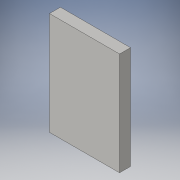
# Autodesk Inventor part: cwbreadboard
Saved by Autodesk Inventor 2016 (Build 200138000, 138)
## iProperties
Created: 2017-08-31
Part Number: cwbreadboard
Material: Generic
Document SubType Name: Modeling
Designer: student
Density: 1 g/cm^3
Appearance: Default
Author: student
Autodesk Inventor part; units mm, degrees
ref_plane "YZ Plane" through (0, 0, 0) normal (1, 0, 0) x (0, 1, 0)
ref_plane "XZ Plane" through (0, 0, 0) normal (0, 1, 0) x (-1, 0, 0)
ref_plane "XY Plane" through (0, 0, 0) normal (0, 0, 1) x (1, 0, 0)
sketch "Sketch1" plane through (0, 0, 0) normal (0, 0, 1) x (1, 0, 0)
  line L0 (-27.6225, -40.5638) -> (27.6225, -40.5638)
  line L1 (27.6225, -40.5638) -> (27.6225, 40.5638)
  line L2 (27.6225, 40.5638) -> (-27.6225, 40.5638)
  line L3 (-27.6225, 40.5638) -> (-27.6225, -40.5638)
  point P0 (0, 0)
  dimension "d0" = 55.245
  dimension "d1" = 81.1276
  constraints: 8 end point, 2 parallel, 1 horizontal, 1 perpendicular
  measures "d0" distance of L2.end L1.end
  measures "d1" distance of L2.end L0.start
extrude "Extrusion1" add sketch "Sketch1" along normal blind 8.636
body "Solid1"
